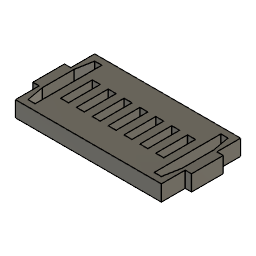
horizontal inlay (Autodesk Fusion 360 design; units mm, degrees)
Autodesk Fusion 360 part; units mm, degrees
sketch "Sketch1" plane through (0, 0, 0) normal (0, 0, 1) x (1, 0, 0)
  line L0 (23, 25) -> (0, 25)
  line L1 (0, 25) -> (0, 0)
  line L2 (0, 0) -> (23, 0)
  line L3 (25, 7.5) -> (25, 17.5)
  line L4 (25, 12.5) -> (0, 12.5) construction
  line L5 (25, 7.5) -> (23, 7.5)
  line L6 (23, 7.5) -> (23, 0)
  line L7 (25, 17.5) -> (23, 17.5)
  line L8 (23, 17.5) -> (23, 25)
  line L9 (21, 23) -> (18.75, 23)
  line L10 (18.75, 23) -> (18.75, 2)
  line L11 (18.75, 2) -> (21, 2)
  line L12 (21, 2) -> (22, 7.5)
  line L13 (22, 17.5) -> (21, 23)
  line L14 (16.25, 17.5) -> (13.75, 17.5)
  line L15 (13.75, 17.5) -> (13.75, 7.5)
  line L16 (13.75, 7.5) -> (16.25, 7.5)
  line L17 (16.25, 7.5) -> (16.25, 17.5)
  line L18 (22, 7.5) -> (22, 17.5)
  point P0 (25, 12.5)
  point P1 (18.75, 12.5)
  point P2 (16.25, 12.5)
  point P3 (22, 12.5)
  dimension "d6" = 2
  dimension "d7" = 1
  dimension "d8" = 2
  dimension "d9" = 10
  dimension "d10" = 25
  dimension "d11" = 2
  dimension "d13" = 2.5
  dimension "d14" = 2.5
  dimension "d24" = 23
  dimension "d25" = 10
  dimension "d26" = 6.25
  constraint midpoint L1 L4.end
  constraint coincident L3 P0
  constraint midpoint L3 P0
  constraint coincident L4 P0
  constraint midpoint L10 P1
  constraint coincident L4 P1
  constraint midpoint L17 P2
  constraint coincident L4 P2
  constraint coincident L1.end L2.start
  constraint vertical L1
  constraint horizontal L0
  constraint vertical L6
  constraint horizontal L5
  constraint vertical L3
  constraint horizontal L7
  constraint vertical L8
  constraint vertical L15
  constraint horizontal L14
  constraint vertical L17
  constraint horizontal L16
  constraint horizontal L11
  constraint horizontal L4
  constraint vertical L9.start L11.end
  constraint vertical L5.end L7.end
  constraint midpoint L18 P3
  constraint coincident L4 P3
  constraint vertical L18
  constraint coincident L7 L13.start
  measures "d6" distance of L3.start L5.end
  measures "d7" distance of L8 L12.end
  measures "d8" distance of L8 L9.start
  measures "d9" distance of L3.start L3.end
  measures "d10" distance of L0 L2
  measures "d11" distance of L0 L9
  measures "d13" distance of L10 L17
  measures "d14" distance of L14.start L14.end
  measures "d24" distance of L0.end L0.start
  measures "d25" distance of L14.end L15.end
  measures "d26" distance of L3 L10
extrude "Extrude1" add sketch "Sketch1" along normal mid plane 5 contours L0 L1 L2 L3 L5 L6 L7 L8 | L14 L15 L16 L17
extrude "Extrude2" cut sketch "Sketch1" along normal through all and the other way through all contours L14 L15 L16 L17
pattern_linear "R-Pattern1" count 11 spacing 5 along (-1, 0, 0) of "Extrude2"
mirror "Mirror1" about plane through (0, 25, 0) normal (-1, 0, 0) of bodies 1 merged
equation "unit_size = 25 mm"
equation "wall_thickness = 2 mm"
equation "column_units = 2"
equation "d6 = wall_thickness"
equation "d24 = unit_size * column_units / 2 - wall_thickness"
equation "d25 = 2 * unit_size / 5"
